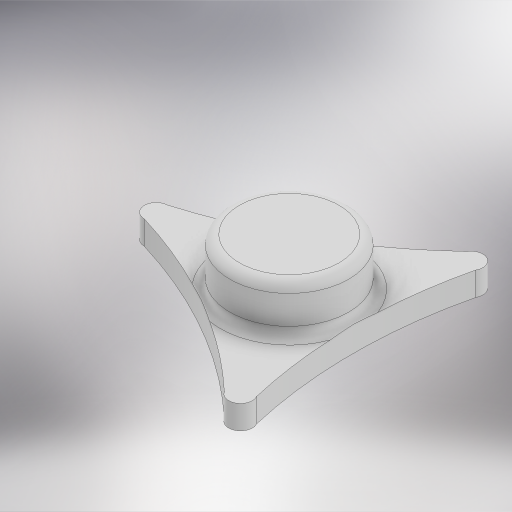
# Autodesk Inventor part: Portaplanetas
Saved by Autodesk Inventor 2024.3 (Build 283343000, 343)
## iProperties
Created: 2025-03-05
Part Number: Portaplanetas
Material: Generic
Document SubType Name: Modeling
Designer: danie
Density: 1 g/cm^3
Appearance: Default
Author: danie
Autodesk Inventor part; units mm, degrees
ref_plane "YZ Plane" through (0, 0, 0) normal (1, 0, 0) x (0, 1, 0)
ref_plane "XZ Plane" through (0, 0, 0) normal (0, 1, 0) x (-1, 0, 0)
ref_plane "XY Plane" through (0, 0, 0) normal (0, 0, 1) x (1, 0, 0)
sketch "Sketch1" plane through (0, 0, 0) normal (0, 1, 0) x (-1, 0, 0)
  circle A0 centre (0, 0) radius 12.5
  circle A1 centre (0, 0) radius 12
  dimension "d0" = 25
  dimension "d1" = 24
  constraints: 2 centre point, 2 coincident
  measures "d0" diameter of A0
  measures "d1" diameter of A1
extrude "Extrusion1" add sketch "Sketch1" along normal blind 10 contours A0 | A1
sketch "Sketch2" plane through (0, 0, 0) normal (0, -1, 0) x (1, 0, 0)
  line L0 (0, 0) -> (-28, 0)
  line L1 (0, 0) -> (14, -24.2487)
  line L2 (0, 0) -> (14, 24.2487)
  line L3 (0, 2.5) -> (-28, 2.5)
  line L4 (0, -2.5) -> (-28, -2.5)
  arc A0 (-28, 2.5) -> (-28, -2.5) centre (-28, 0) ccw
  line L5 (2.1651, 1.25) -> (16.1651, -22.9987)
  line L6 (-2.1651, -1.25) -> (11.8349, -25.4987)
  arc A1 (11.8349, -25.4987) -> (16.1651, -22.9987) centre (14, -24.2487) ccw
  line L7 (-2.1651, 1.25) -> (11.8349, 25.4987)
  line L8 (2.1651, -1.25) -> (16.1651, 22.9987)
  arc A2 (16.1651, 22.9987) -> (11.8349, 25.4987) centre (14, 24.2487) ccw
  arc A3 (11.8349, -25.4987) -> (-28, -2.5) centre (-56.7422, -98.2804) ccw
  arc A4 (16.1651, 22.9987) -> (16.1651, -22.9987) centre (113.4844, 0) ccw
  arc A5 (-28, 2.5) -> (11.8349, 25.4987) centre (-56.7422, 98.2804) ccw
  dimension "d4" = 28
  dimension "d7" = 360
  dimension "d9" = 2.5
  dimension "d10" = 2.5
  dimension "d11" = 2.5
  dimension "d14" = 360
  dimension "d16" = 100
  dimension "d19" = 360
  constraints: 18 end point, 12 point on circle, 6 centre point, 2 coincident, 2 parallel, 1 horizontal, 46 other
  measures "d4" distance of L0.start L0.end
  measures "d9" distance between parallel lines of L0 L3
  measures "d10" distance between parallel lines of L0 L4
  measures "d11" radius of A0
  measures "d16" radius of A3
extrude "Extrusion2" add sketch "Sketch2" along normal blind 5
fillet "Fillet1" radius 2 2 edges at (12.5, 0, 0) (12.5, 10, 0)
body "Solid1"
